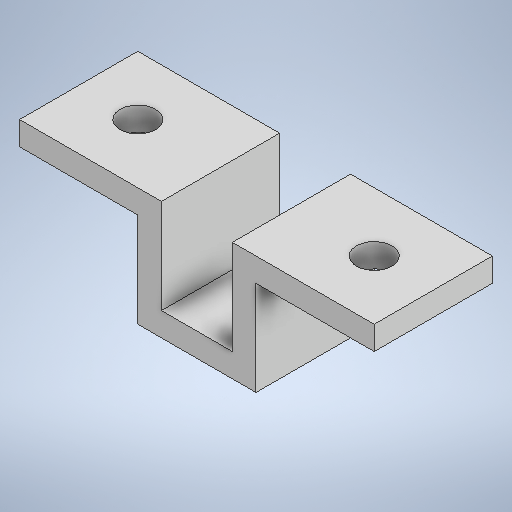
# Autodesk Inventor part: CAM_HOLD
Saved by Autodesk Inventor 2025.3 (Build 293356030, 356C)
## iProperties
Created: 2026-06-30
Part Number: CAM_HOLD
Material: Generic
Document SubType Name: Modeling
Designer: user
Density: 1 g/cm^3
Appearance: Default
Author: user
Autodesk Inventor part; units mm, degrees
ref_plane "YZ Plane" through (0, 0, 0) normal (1, 0, 0) x (0, 1, 0)
ref_plane "XZ Plane" through (0, 0, 0) normal (0, 1, 0) x (-1, 0, 0)
ref_plane "XY Plane" through (0, 0, 0) normal (0, 0, 1) x (1, 0, 0)
sketch "Sketch1" plane through (0, 0, 0) normal (0, 0, 1) x (1, 0, 0)
  line L0 (0, 0) -> (10, 0)
  line L1 (10, 0) -> (10, 8)
  line L2 (0, 8) -> (0, 0)
  line L3 (8, 10) -> (8, 2)
  line L4 (8, 2) -> (2, 2)
  line L5 (2, 2) -> (2, 8)
  line L6 (0, 8) -> (-10, 8)
  line L7 (-10, 8) -> (-10, 10)
  line L8 (10, 8) -> (20, 8)
  line L9 (20, 8) -> (20, 10)
  line L10 (2, 8) -> (2, 10)
  line L11 (-10, 10) -> (2, 10)
  line L12 (8, 10) -> (20, 10)
  line L13 (10, 10) -> (8, 10)
  line L14 (2, 10) -> (0, 10)
  dimension "d3" = 10
  dimension "d4" = 10
  constraints: 30 end point, 6 perpendicular, 4 parallel, 1 horizontal
  measures "d3" distance between parallel lines of L2 L7
  measures "d4" distance of L1.end L8.end
extrude "Extrusion1" add sketch "Sketch1" along normal blind 10
sketch "Sketch2" plane through (-10, 10, 0) normal (0, 1, 0) x (1, 0, 0)
  line L0 (12, -10) -> (0, -10) projected
  line L1 (0, 0) -> (0, -10) projected
  line L2 (30, 0) -> (18, 0) projected
  line L3 (30, 0) -> (30, -10) projected
  point P0 (10, 0)
  point P1 (5, -5)
  point P2 (25, -5)
  dimension "d14" = 5
  dimension "d15" = 5
  dimension "d16" = 5
  dimension "d17" = 5
  measures "d14" distance from line of L0 point (5, -5)
  measures "d15" distance from line of L1 point (5, -5)
  measures "d16" distance from line of L2 point (25, -5)
  measures "d17" distance from line of L3 point (25, -5)
hole "Hole1" at (-5, 10, 5) at (15, 10, 5) direction (0, -1, 0) diameter 3 end through all
body "Solid1"
